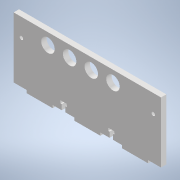
# Autodesk Inventor part: caja_2_Lateral
Saved by Autodesk Inventor 2022 (Build 260153000, 153)
## iProperties
Created: 2022-03-11
Part Number: caja_2_Lateral
Material: Generic
Document SubType Name: Modeling
Designer: katha
Density: 1 g/cm^3
Appearance: Default
Author: katha
Autodesk Inventor part; units mm, degrees
ref_plane "YZ Plane" through (0, 0, 0) normal (1, 0, 0) x (0, 1, 0)
ref_plane "XZ Plane" through (0, 0, 0) normal (0, 1, 0) x (-1, 0, 0)
ref_plane "XY Plane" through (0, 0, 0) normal (0, 0, 1) x (1, 0, 0)
sketch "Sketch1" plane through (0, 0, 0) normal (0, 0, 1) x (1, 0, 0)
  circle A0 centre (-76, 20.6153) radius 2 projected
  circle A1 centre (76, 20.6157) radius 2 projected
  line L0 (25.6401, -28.4) -> (25.6401, -22.3) projected
  line L1 (25.6401, -22.3) -> (24.1401, -22.3) projected
  line L2 (24.1401, -22.3) -> (24.1401, -19.1) projected
  line L3 (24.1401, -19.1) -> (31.1401, -19.1) projected
  line L4 (31.1401, -19.1) -> (31.1401, -22.3) projected
  line L5 (31.1401, -22.3) -> (29.6401, -22.3) projected
  line L6 (29.6401, -22.3) -> (29.6401, -28.4) projected
  line L7 (29.6401, -28.4) -> (40.1868, -28.4) projected
  line L8 (40.1868, -28.4) -> (40.1868, -31.6) projected
  line L9 (40.1868, -31.6) -> (70.1868, -31.6) projected
  line L10 (70.1868, -31.6) -> (70.1868, -28.4) projected
  line L11 (70.1868, -28.4) -> (85, -28.4) projected
  line L12 (85, -28.4) -> (85, 31.6) projected
  line L13 (85, 31.6) -> (70.6157, 31.6) projected
  arc A2 (56.2026, 31.6) -> (70.6157, 31.6) centre (63.4091, 28.6157) ccw projected
  line L14 (56.2026, 31.6) -> (33.0157, 31.6) projected
  arc A3 (18.603, 31.6) -> (33.0157, 31.6) centre (25.8094, 28.6153) ccw projected
  line L15 (18.603, 31.6) -> (-2.4569, 31.6) projected
  arc A4 (-16.8696, 31.6) -> (-2.4569, 31.6) centre (-9.6632, 28.6153) ccw projected
  line L16 (-16.8696, 31.6) -> (-38.2294, 31.6) projected
  arc A5 (-52.6422, 31.6) -> (-38.2294, 31.6) centre (-45.4358, 28.6153) ccw projected
  line L17 (-52.6422, 31.6) -> (-85, 31.6) projected
  line L18 (-85, 31.6) -> (-85, -28.4) projected
  line L19 (-85, -28.4) -> (-70, -28.4) projected
  line L20 (-70, -28.4) -> (-70, -31.6) projected
  line L21 (-70, -31.6) -> (-40, -31.6) projected
  line L22 (-40, -31.6) -> (-40, -28.4) projected
  line L23 (-40, -28.4) -> (-29.4533, -28.4) projected
  line L24 (-29.4533, -28.4) -> (-29.4533, -22.3) projected
  line L25 (-29.4533, -22.3) -> (-30.9533, -22.3) projected
  line L26 (-30.9533, -22.3) -> (-30.9533, -19.1) projected
  line L27 (-30.9533, -19.1) -> (-23.9533, -19.1) projected
  line L28 (-23.9533, -19.1) -> (-23.9533, -22.3) projected
  line L29 (-23.9533, -22.3) -> (-25.4533, -22.3) projected
  line L30 (-25.4533, -22.3) -> (-25.4533, -28.4) projected
  line L31 (-25.4533, -28.4) -> (-14.9066, -28.4) projected
  line L32 (-14.9066, -28.4) -> (-14.9066, -31.6) projected
  line L33 (-14.9066, -31.6) -> (15.0934, -31.6) projected
  line L34 (15.0934, -31.6) -> (15.0934, -28.4) projected
  line L35 (15.0934, -28.4) -> (25.6401, -28.4) projected
  circle A6 centre (-45.4358, 28.6153) radius 7.8
  circle A7 centre (-20.4358, 28.6153) radius 7.8
  circle A8 centre (4.5642, 28.6153) radius 7.8
  circle A9 centre (29.5642, 28.6153) radius 7.8
  line L36 (85, -28.4) -> (85, 41.6)
  line L37 (85, 41.6) -> (-85, 41.6)
  line L38 (-85, 41.6) -> (-85, -28.4)
  line L39 (-85, -28.4) -> (-70, -28.4)
  line L40 (-70, -28.4) -> (-70, -31.6)
  line L41 (-70, -31.6) -> (-40, -31.6)
  line L42 (-40, -31.6) -> (-40, -28.4)
  line L43 (-40, -28.4) -> (-29.4533, -28.4)
  line L44 (-29.4533, -28.4) -> (-29.4533, -22.3)
  line L45 (-29.4533, -22.3) -> (-30.9533, -22.3)
  line L46 (-30.9533, -22.3) -> (-30.9533, -19.1)
  line L47 (-30.9533, -19.1) -> (-23.9533, -19.1)
  line L48 (-23.9533, -19.1) -> (-23.9533, -22.3)
  line L49 (-23.9533, -22.3) -> (-25.4533, -22.3)
  line L50 (-25.4533, -22.3) -> (-25.4533, -28.4)
  line L51 (-25.4533, -28.4) -> (-14.9066, -28.4)
  line L52 (-14.9066, -28.4) -> (-14.9066, -31.6)
  line L53 (-14.9066, -31.6) -> (15.0934, -31.6)
  line L54 (15.0934, -31.6) -> (15.0934, -28.4)
  line L55 (15.0934, -28.4) -> (25.6401, -28.4)
  line L56 (25.6401, -28.4) -> (25.6401, -22.3)
  line L57 (25.6401, -22.3) -> (24.1401, -22.3)
  line L58 (24.1401, -22.3) -> (24.1401, -19.1)
  line L59 (24.1401, -19.1) -> (31.1401, -19.1)
  line L60 (31.1401, -19.1) -> (31.1401, -22.3)
  line L61 (31.1401, -22.3) -> (29.6401, -22.3)
  line L62 (29.6401, -22.3) -> (29.6401, -28.4)
  line L63 (29.6401, -28.4) -> (40.1868, -28.4)
  line L64 (40.1868, -28.4) -> (40.1868, -31.6)
  line L65 (40.1868, -31.6) -> (70.1868, -31.6)
  line L66 (70.1868, -31.6) -> (70.1868, -28.4)
  line L67 (85, -28.4) -> (70.1868, -28.4)
  circle A10 centre (76, 20.6157) radius 2
  circle A11 centre (-76, 20.6153) radius 2
  point P0 (0, 0)
  dimension "d0" = 25
  dimension "d1" = 25
  dimension "d2" = 25
  dimension "d3" = 70
  constraints: 64 end point, 19 collinear, 11 perpendicular, 5 centre point, 3 coincident, 3 horizontal alignment, 2 concentric, 2 equal radius, 1 parallel, 1 point on line, 4 other
  measures "d0" distance of A5.centre A7.centre
  measures "d1" distance of A8.centre A7.centre
  measures "d2" distance of A9.centre A8.centre
  measures "d3" distance of L11.end L36.end
extrude "Extrusion1" add sketch "Sketch1" along normal blind 6.2 contours L35 L34 L33 L32 L31 L30 L29 L28 L27 L26 L25 L24 L23 L22 L21 L20 L19 L18 L17 A5 L16 A7 A4 A8 L15 A3 A9 L14 A2 L13 L12 L11 L10 L9 L8 L7 L6 L5 L4 L3 L2 L1 L0 | L13 A2 L14 A9 A3 L15 A8 A4 A7 L16 A6 L17 L38 L37 L36
body "Solid1"
